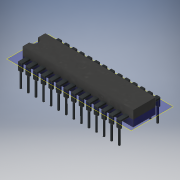
# Autodesk Inventor part: K572ПВ4
Saved by Autodesk Inventor 2019 (Build 230136000, 136)
## iProperties
Created: 2020-03-31
Part Number: K572ПВ4
Material: Generic
Document SubType Name: Modeling
Designer: user
Density: 1 g/cm^3
Appearance: Default
Author: user
Autodesk Inventor part; units mm, degrees
ref_plane "YZ Plane" through (0, 0, 0) normal (1, 0, 0) x (0, 1, 0)
ref_plane "XZ Plane" through (0, 0, 0) normal (0, 1, 0) x (-1, 0, 0)
ref_plane "XY Plane" through (0, 0, 0) normal (0, 0, 1) x (1, 0, 0)
sketch "Sketch1" plane through (0, 0, 0) normal (0, 1, 0) x (-1, 0, 0)
  line L0 (0, 0) -> (37, 0)
  line L1 (37, 0) -> (37, -7.5)
  line L2 (37, -7.5) -> (0, -7.5)
  line L3 (0, -7.5) -> (0, 0)
  dimension "d0" = 37
  dimension "d1" = 7.5
  constraints: 8 end point, 2 parallel, 1 horizontal, 1 perpendicular
  measures "d0" distance of L1.end L2.end
  measures "d1" distance between parallel lines of L0 L2
extrude "Extrusion1" add sketch "Sketch1" along normal blind 5
sketch "Sketch2" plane through (-37, 0, 0) normal (0, 0, 1) x (1, 0, 0)
  line L0 (37, 0) -> (37, 5) projected
  line L1 (2.6, 2.2) -> (1.4, 2.2)
  line L2 (1.4, 2.2) -> (1.4, 2.8)
  line L3 (1.4, 2.8) -> (2.6, 2.8)
  line L4 (2.6, 2.8) -> (2.6, 2.2)
  line L5 (2.6, 2.2) -> (1.4, 2.8) construction
  line L6 (1.4, 2.2) -> (2.6, 2.8) construction
  line L7 (5.14, 2.2) -> (3.94, 2.2)
  line L8 (3.94, 2.2) -> (3.94, 2.8)
  line L9 (3.94, 2.8) -> (5.14, 2.8)
  line L10 (5.14, 2.8) -> (5.14, 2.2)
  line L11 (7.68, 2.2) -> (6.48, 2.2)
  line L12 (6.48, 2.2) -> (6.48, 2.8)
  line L13 (6.48, 2.8) -> (7.68, 2.8)
  line L14 (7.68, 2.8) -> (7.68, 2.2)
  line L15 (10.22, 2.2) -> (9.02, 2.2)
  line L16 (9.02, 2.2) -> (9.02, 2.8)
  line L17 (9.02, 2.8) -> (10.22, 2.8)
  line L18 (10.22, 2.8) -> (10.22, 2.2)
  line L19 (12.76, 2.2) -> (11.56, 2.2)
  line L20 (11.56, 2.2) -> (11.56, 2.8)
  line L21 (11.56, 2.8) -> (12.76, 2.8)
  line L22 (12.76, 2.8) -> (12.76, 2.2)
  line L23 (15.3, 2.2) -> (14.1, 2.2)
  line L24 (14.1, 2.2) -> (14.1, 2.8)
  line L25 (14.1, 2.8) -> (15.3, 2.8)
  line L26 (15.3, 2.8) -> (15.3, 2.2)
  line L27 (17.84, 2.2) -> (16.64, 2.2)
  line L28 (16.64, 2.2) -> (16.64, 2.8)
  line L29 (16.64, 2.8) -> (17.84, 2.8)
  line L30 (17.84, 2.8) -> (17.84, 2.2)
  line L31 (20.38, 2.2) -> (19.18, 2.2)
  line L32 (19.18, 2.2) -> (19.18, 2.8)
  line L33 (19.18, 2.8) -> (20.38, 2.8)
  line L34 (20.38, 2.8) -> (20.38, 2.2)
  line L35 (22.92, 2.2) -> (21.72, 2.2)
  line L36 (21.72, 2.2) -> (21.72, 2.8)
  line L37 (21.72, 2.8) -> (22.92, 2.8)
  line L38 (22.92, 2.8) -> (22.92, 2.2)
  line L39 (25.46, 2.2) -> (24.26, 2.2)
  line L40 (24.26, 2.2) -> (24.26, 2.8)
  line L41 (24.26, 2.8) -> (25.46, 2.8)
  line L42 (25.46, 2.8) -> (25.46, 2.2)
  line L43 (28, 2.2) -> (26.8, 2.2)
  line L44 (26.8, 2.2) -> (26.8, 2.8)
  line L45 (26.8, 2.8) -> (28, 2.8)
  line L46 (28, 2.8) -> (28, 2.2)
  line L47 (30.54, 2.2) -> (29.34, 2.2)
  line L48 (29.34, 2.2) -> (29.34, 2.8)
  line L49 (29.34, 2.8) -> (30.54, 2.8)
  line L50 (30.54, 2.8) -> (30.54, 2.2)
  line L51 (33.08, 2.2) -> (31.88, 2.2)
  line L52 (31.88, 2.2) -> (31.88, 2.8)
  line L53 (31.88, 2.8) -> (33.08, 2.8)
  line L54 (33.08, 2.8) -> (33.08, 2.2)
  line L55 (35.62, 2.2) -> (34.42, 2.2)
  line L56 (34.42, 2.2) -> (34.42, 2.8)
  line L57 (34.42, 2.8) -> (35.62, 2.8)
  line L58 (35.62, 2.8) -> (35.62, 2.2)
  dimension "d19" = 1.2
  dimension "d20" = 0.6
  dimension "d21" = 1.2
  dimension "d22" = 0.6
  dimension "d23" = 1.2
  dimension "d25" = 1.2
  dimension "d27" = 1.2
  dimension "d28" = 0.6
  dimension "d29" = 1.2
  dimension "d31" = 1.2
  dimension "d32" = 0.6
  dimension "d33" = 1.2
  dimension "d34" = 0.6
  dimension "d35" = 1.2
  dimension "d36" = 0.6
  dimension "d37" = 1.2
  dimension "d38" = 0.6
  dimension "d39" = 1.2
  dimension "d40" = 0.6
  dimension "d41" = 1.2
  dimension "d42" = 0.6
  dimension "d43" = 1.2
  dimension "d44" = 0.6
  dimension "d45" = 1.2
  dimension "d46" = 0.6
  constraints: 116 end point, 28 parallel, 14 horizontal, 14 perpendicular
  measures "d19" distance of L2.end L3.end
  measures "d20" distance of L1.end L2.end
  measures "d21" distance of L9.start L9.end
  measures "d22" distance of L8.start L9.start
  measures "d23" distance of L13.start L13.end
  measures "d25" distance of L17.start L17.end
  measures "d27" distance of L21.start L21.end
  measures "d28" distance of L20.start L21.start
  measures "d29" distance of L25.start L25.end
  measures "d31" distance of L29.start L29.end
  measures "d32" distance of L28.start L29.start
  measures "d33" distance of L33.start L33.end
  measures "d34" distance of L32.start L33.start
  measures "d35" distance of L37.start L37.end
  measures "d36" distance of L36.start L37.start
  measures "d37" distance of L41.start L41.end
  measures "d38" distance of L40.start L41.start
  measures "d39" distance of L45.start L45.end
  measures "d40" distance of L44.start L45.start
  measures "d41" distance of L49.start L49.end
  measures "d42" distance of L48.start L49.start
  measures "d43" distance of L53.start L53.end
  measures "d44" distance of L52.start L53.start
  measures "d45" distance of L57.start L57.end
  measures "d46" distance of L56.start L57.start
extrude "Extrusion2" add sketch "Sketch2" along normal blind 3
sketch "Sketch3" plane through (0, 0, -7.5) normal (0, 0, -1) x (-1, 0, 0)
  line L0 (0, 0) -> (0, 5) projected
  line L1 (1.4, 2.2) -> (2.6, 2.2)
  line L2 (2.6, 2.2) -> (2.6, 2.8)
  line L3 (2.6, 2.8) -> (1.4, 2.8)
  line L4 (1.4, 2.8) -> (1.4, 2.2)
  line L5 (1.4, 2.2) -> (2.6, 2.8) construction
  line L6 (2.6, 2.2) -> (1.4, 2.8) construction
  line L7 (3.94, 2.2) -> (5.14, 2.2)
  line L8 (5.14, 2.2) -> (5.14, 2.8)
  line L9 (5.14, 2.8) -> (3.94, 2.8)
  line L10 (3.94, 2.8) -> (3.94, 2.2)
  line L11 (6.48, 2.2) -> (7.68, 2.2)
  line L12 (7.68, 2.2) -> (7.68, 2.8)
  line L13 (7.68, 2.8) -> (6.48, 2.8)
  line L14 (6.48, 2.8) -> (6.48, 2.2)
  line L15 (9.02, 2.2) -> (10.22, 2.2)
  line L16 (10.22, 2.2) -> (10.22, 2.8)
  line L17 (10.22, 2.8) -> (9.02, 2.8)
  line L18 (9.02, 2.8) -> (9.02, 2.2)
  line L19 (11.56, 2.2) -> (12.76, 2.2)
  line L20 (12.76, 2.2) -> (12.76, 2.8)
  line L21 (12.76, 2.8) -> (11.56, 2.8)
  line L22 (11.56, 2.8) -> (11.56, 2.2)
  line L23 (14.1, 2.2) -> (15.3, 2.2)
  line L24 (15.3, 2.2) -> (15.3, 2.8)
  line L25 (15.3, 2.8) -> (14.1, 2.8)
  line L26 (14.1, 2.8) -> (14.1, 2.2)
  line L27 (16.64, 2.2) -> (17.84, 2.2)
  line L28 (17.84, 2.2) -> (17.84, 2.8)
  line L29 (17.84, 2.8) -> (16.64, 2.8)
  line L30 (16.64, 2.8) -> (16.64, 2.2)
  line L31 (16.64, 2.8) -> (16.64, 2.2)
  line L32 (17.84, 2.8) -> (16.64, 2.8)
  line L33 (17.84, 2.2) -> (17.84, 2.8)
  line L34 (16.64, 2.2) -> (17.84, 2.2)
  line L35 (19.18, 2.8) -> (19.18, 2.2)
  line L36 (20.38, 2.8) -> (19.18, 2.8)
  line L37 (20.38, 2.2) -> (20.38, 2.8)
  line L38 (19.18, 2.2) -> (20.38, 2.2)
  line L39 (21.72, 2.8) -> (21.72, 2.2)
  line L40 (22.92, 2.8) -> (21.72, 2.8)
  line L41 (22.92, 2.2) -> (22.92, 2.8)
  line L42 (21.72, 2.2) -> (22.92, 2.2)
  line L43 (24.26, 2.8) -> (24.26, 2.2)
  line L44 (25.46, 2.8) -> (24.26, 2.8)
  line L45 (25.46, 2.2) -> (25.46, 2.8)
  line L46 (24.26, 2.2) -> (25.46, 2.2)
  line L47 (26.8, 2.8) -> (26.8, 2.2)
  line L48 (28, 2.8) -> (26.8, 2.8)
  line L49 (28, 2.2) -> (28, 2.8)
  line L50 (26.8, 2.2) -> (28, 2.2)
  line L51 (29.34, 2.8) -> (29.34, 2.2)
  line L52 (30.54, 2.8) -> (29.34, 2.8)
  line L53 (30.54, 2.2) -> (30.54, 2.8)
  line L54 (29.34, 2.2) -> (30.54, 2.2)
  line L55 (31.88, 2.8) -> (31.88, 2.2)
  line L56 (33.08, 2.8) -> (31.88, 2.8)
  line L57 (33.08, 2.2) -> (33.08, 2.8)
  line L58 (31.88, 2.2) -> (33.08, 2.2)
  line L59 (34.42, 2.8) -> (34.42, 2.2)
  line L60 (35.62, 2.8) -> (34.42, 2.8)
  line L61 (35.62, 2.2) -> (35.62, 2.8)
  line L62 (34.42, 2.2) -> (35.62, 2.2)
  dimension "d63" = 1.2
  dimension "d64" = 0.6
  dimension "d65" = 1.2
  dimension "d66" = 0.6
  dimension "d67" = 1.2
  dimension "d68" = 0.6
  dimension "d69" = 1.2
  dimension "d70" = 0.6
  dimension "d71" = 1.2
  dimension "d72" = 0.6
  dimension "d73" = 1.2
  dimension "d74" = 0.6
  dimension "d75" = 1.2
  dimension "d76" = 0.6
  dimension "d77" = 1.2
  dimension "d78" = 0.6
  dimension "d79" = 1.2
  dimension "d80" = 0.6
  dimension "d81" = 1.2
  dimension "d82" = 0.6
  dimension "d83" = 1.2
  dimension "d84" = 0.6
  dimension "d85" = 1.2
  dimension "d86" = 0.6
  dimension "d87" = 1.2
  dimension "d88" = 0.6
  dimension "d89" = 1.2
  dimension "d90" = 0.6
  dimension "d91" = 1.2
  dimension "d92" = 0.6
  constraints: 124 end point, 30 parallel, 15 horizontal, 15 perpendicular
  measures "d63" distance of L3.end L2.end
  measures "d64" distance between parallel lines of L1 L3
  measures "d65" distance of L10.start L9.start
  measures "d66" distance between parallel lines of L7 L9
  measures "d67" distance of L14.start L13.start
  measures "d68" distance between parallel lines of L11 L13
  measures "d69" distance of L18.start L17.start
  measures "d70" distance between parallel lines of L15 L17
  measures "d71" distance of L22.start L21.start
  measures "d72" distance between parallel lines of L19 L21
  measures "d73" distance of L26.start L25.start
  measures "d74" distance between parallel lines of L23 L25
  measures "d75" distance of L30.start L29.start
  measures "d76" distance between parallel lines of L27 L29
  measures "d77" distance of L32.end L32.start
  measures "d78" distance between parallel lines of L34 L32
  measures "d79" distance of L36.end L36.start
  measures "d80" distance between parallel lines of L38 L36
  measures "d81" distance of L40.end L40.start
  measures "d82" distance between parallel lines of L42 L40
  measures "d83" distance of L44.end L44.start
  measures "d84" distance between parallel lines of L46 L44
  measures "d85" distance of L48.end L48.start
  measures "d86" distance between parallel lines of L50 L48
  measures "d87" distance of L52.end L52.start
  measures "d88" distance between parallel lines of L54 L52
  measures "d89" distance of L56.end L56.start
  measures "d90" distance between parallel lines of L58 L56
  measures "d91" distance of L60.end L60.start
  measures "d92" distance between parallel lines of L62 L60
extrude "Extrusion3" add sketch "Sketch3" along normal blind 3
ref_plane "Work Plane2" through (-35.6, 2.2, 3) normal (0, -1, 0) x (1, 0, 0)
sketch "Sketch6" plane through (-35.6, 2.2, 3) normal (0, -1, 0) x (1, 0, 0)
  line L0 (0, 0) -> (1.2, 0)
  line L1 (1.2, 0) -> (1.2, -0.6)
  line L2 (1.2, -0.6) -> (0, -0.6)
  line L3 (0, -0.6) -> (0, 0)
  line L4 (2.5041, 0) -> (3.7041, 0)
  line L5 (3.7041, 0) -> (3.7041, -0.6)
  line L6 (3.7041, -0.6) -> (2.5041, -0.6)
  line L7 (2.5041, -0.6) -> (2.5041, 0)
  line L8 (5.0877, 0) -> (6.2877, 0)
  line L9 (6.2877, 0) -> (6.2877, -0.6)
  line L10 (6.2877, -0.6) -> (5.0877, -0.6)
  line L11 (5.0877, -0.6) -> (5.0877, 0)
  line L12 (7.6344, 0) -> (8.8344, 0)
  line L13 (8.8344, 0) -> (8.8344, -0.6)
  line L14 (8.8344, -0.6) -> (7.6344, -0.6)
  line L15 (7.6344, -0.6) -> (7.6344, 0)
  line L16 (10.1527, 0) -> (11.3527, 0)
  line L17 (11.3527, 0) -> (11.3527, -0.6)
  line L18 (11.3527, -0.6) -> (10.1527, -0.6)
  line L19 (10.1527, -0.6) -> (10.1527, 0)
  line L20 (12.7058, 0) -> (13.9058, 0)
  line L21 (13.9058, 0) -> (13.9058, -0.6)
  line L22 (13.9058, -0.6) -> (12.7058, -0.6)
  line L23 (12.7058, -0.6) -> (12.7058, 0)
  line L24 (15.2415, 0) -> (16.4415, 0)
  line L25 (16.4415, 0) -> (16.4415, -0.6)
  line L26 (16.4415, -0.6) -> (15.2415, -0.6)
  line L27 (15.2415, -0.6) -> (15.2415, 0)
  line L28 (17.7945, 0) -> (18.9945, 0)
  line L29 (18.9945, 0) -> (18.9945, -0.6)
  line L30 (18.9945, -0.6) -> (17.7945, -0.6)
  line L31 (17.7945, -0.6) -> (17.7945, 0)
  line L32 (20.3302, 0) -> (21.5302, 0)
  line L33 (21.5302, 0) -> (21.5302, -0.6)
  line L34 (21.5302, -0.6) -> (20.3302, -0.6)
  line L35 (20.3302, -0.6) -> (20.3302, 0)
  line L36 (22.8658, 0) -> (24.0658, 0)
  line L37 (24.0658, 0) -> (24.0658, -0.6)
  line L38 (24.0658, -0.6) -> (22.8658, -0.6)
  line L39 (22.8658, -0.6) -> (22.8658, 0)
  line L40 (-0.0033, -12.9) -> (1.1967, -12.9)
  line L41 (1.1967, -12.9) -> (1.1967, -13.5)
  line L42 (1.1967, -13.5) -> (-0.0033, -13.5)
  line L43 (-0.0033, -13.5) -> (-0.0033, -12.9)
  line L44 (25.3789, 0) -> (26.5789, 0)
  line L45 (26.5789, 0) -> (26.5789, -0.6)
  line L46 (26.5789, -0.6) -> (25.3789, -0.6)
  line L47 (25.3789, -0.6) -> (25.3789, 0)
  line L48 (27.932, 0) -> (29.132, 0)
  line L49 (29.132, 0) -> (29.132, -0.6)
  line L50 (29.132, -0.6) -> (27.932, -0.6)
  line L51 (27.932, -0.6) -> (27.932, 0)
  line L52 (30.4676, 0) -> (31.6676, 0)
  line L53 (31.6676, 0) -> (31.6676, -0.6)
  line L54 (31.6676, -0.6) -> (30.4676, -0.6)
  line L55 (30.4676, -0.6) -> (30.4676, 0)
  line L56 (33.0033, 0) -> (34.2033, 0)
  line L57 (34.2033, 0) -> (34.2033, -0.6)
  line L58 (34.2033, -0.6) -> (33.0033, -0.6)
  line L59 (33.0033, -0.6) -> (33.0033, 0)
  line L60 (2.5008, -12.9) -> (3.7008, -12.9)
  line L61 (3.7008, -12.9) -> (3.7008, -13.5)
  line L62 (3.7008, -13.5) -> (2.5008, -13.5)
  line L63 (2.5008, -13.5) -> (2.5008, -12.9)
  line L64 (5.0844, -12.9) -> (6.2844, -12.9)
  line L65 (6.2844, -12.9) -> (6.2844, -13.5)
  line L66 (6.2844, -13.5) -> (5.0844, -13.5)
  line L67 (5.0844, -13.5) -> (5.0844, -12.9)
  line L68 (7.6311, -12.9) -> (8.8311, -12.9)
  line L69 (8.8311, -12.9) -> (8.8311, -13.5)
  line L70 (8.8311, -13.5) -> (7.6311, -13.5)
  line L71 (7.6311, -13.5) -> (7.6311, -12.9)
  line L72 (10.1494, -12.9) -> (11.3494, -12.9)
  line L73 (11.3494, -12.9) -> (11.3494, -13.5)
  line L74 (11.3494, -13.5) -> (10.1494, -13.5)
  line L75 (10.1494, -13.5) -> (10.1494, -12.9)
  line L76 (12.7025, -12.9) -> (13.9025, -12.9)
  line L77 (13.9025, -12.9) -> (13.9025, -13.5)
  line L78 (13.9025, -13.5) -> (12.7025, -13.5)
  line L79 (12.7025, -13.5) -> (12.7025, -12.9)
  line L80 (15.2382, -12.9) -> (16.4382, -12.9)
  line L81 (16.4382, -12.9) -> (16.4382, -13.5)
  line L82 (16.4382, -13.5) -> (15.2382, -13.5)
  line L83 (15.2382, -13.5) -> (15.2382, -12.9)
  line L84 (17.7912, -12.9) -> (18.9912, -12.9)
  line L85 (18.9912, -12.9) -> (18.9912, -13.5)
  line L86 (18.9912, -13.5) -> (17.7912, -13.5)
  line L87 (17.7912, -13.5) -> (17.7912, -12.9)
  line L88 (20.3269, -12.9) -> (21.5269, -12.9)
  line L89 (21.5269, -12.9) -> (21.5269, -13.5)
  line L90 (21.5269, -13.5) -> (20.3269, -13.5)
  line L91 (20.3269, -13.5) -> (20.3269, -12.9)
  line L92 (22.8625, -12.9) -> (24.0625, -12.9)
  line L93 (24.0625, -12.9) -> (24.0625, -13.5)
  line L94 (24.0625, -13.5) -> (22.8625, -13.5)
  line L95 (22.8625, -13.5) -> (22.8625, -12.9)
  line L96 (25.3756, -13.5) -> (25.3756, -12.9)
  line L97 (25.3756, -12.9) -> (26.5756, -12.9)
  line L98 (26.5756, -13.5) -> (25.3756, -13.5)
  line L99 (26.5756, -12.9) -> (26.5756, -13.5)
  line L100 (27.9287, -13.5) -> (27.9287, -12.9)
  line L101 (27.9287, -12.9) -> (29.1287, -12.9)
  line L102 (29.1287, -13.5) -> (27.9287, -13.5)
  line L103 (29.1287, -12.9) -> (29.1287, -13.5)
  line L104 (30.4643, -13.5) -> (30.4643, -12.9)
  line L105 (30.4643, -12.9) -> (31.6643, -12.9)
  line L106 (31.6643, -13.5) -> (30.4643, -13.5)
  line L107 (31.6643, -12.9) -> (31.6643, -13.5)
  line L108 (33, -13.5) -> (33, -12.9)
  line L109 (34.2, -12.9) -> (34.2, -13.5)
  line L110 (34.2, -13.5) -> (33, -13.5)
  line L111 (33, -12.9) -> (34.2, -12.9)
  point P0 (35.6, -3)
  dimension "d127" = 1.2
  dimension "d128" = 0.6
  dimension "d129" = 1.2
  dimension "d130" = 0.6
  dimension "d131" = 1.2
  dimension "d132" = 0.6
  dimension "d133" = 1.2
  dimension "d134" = 0.6
  dimension "d135" = 1.2
  dimension "d136" = 0.6
  dimension "d137" = 1.2
  dimension "d138" = 0.6
  dimension "d139" = 1.2
  dimension "d140" = 0.6
  dimension "d141" = 1.2
  dimension "d142" = 0.6
  dimension "d143" = 1.2
  dimension "d144" = 0.6
  dimension "d145" = 1.2
  dimension "d146" = 0.6
  dimension "d152" = 1.2
  dimension "d153" = 0.6
  dimension "d154" = 1.2
  dimension "d155" = 0.6
  dimension "d156" = 1.2
  dimension "d157" = 0.6
  dimension "d158" = 1.2
  dimension "d159" = 0.6
  dimension "d160" = 1.2
  dimension "d161" = 0.6
  dimension "d162" = 1.2
  dimension "d163" = 0.6
  dimension "d164" = 1.2
  dimension "d165" = 0.6
  dimension "d166" = 1.2
  dimension "d167" = 0.6
  dimension "d168" = 1.2
  dimension "d169" = 0.6
  dimension "d170" = 1.2
  dimension "d171" = 0.6
  dimension "d172" = 1.2
  dimension "d173" = 0.6
  dimension "d174" = 1.2
  dimension "d175" = 0.6
  dimension "d176" = 1.2
  dimension "d177" = 0.6
  dimension "d178" = 1.2
  dimension "d179" = 0.6
  dimension "d180" = 1.2
  dimension "d181" = 0.6
  dimension "d182" = 1.2
  dimension "d183" = 0.6
  dimension "d184" = 1.2
  dimension "d185" = 0.6
  dimension "d186" = 1.2
  dimension "d187" = 0.6
  constraints: 224 end point, 56 parallel, 28 horizontal, 28 perpendicular
  measures "d127" distance of L1.end L2.end
  measures "d128" distance of L0.end L1.end
  measures "d129" distance of L5.end L6.end
  measures "d130" distance of L4.end L5.end
  measures "d131" distance of L9.end L10.end
  measures "d132" distance of L8.end L9.end
  measures "d133" distance of L13.end L14.end
  measures "d134" distance of L12.end L13.end
  measures "d135" distance of L17.end L18.end
  measures "d136" distance of L16.end L17.end
  measures "d137" distance of L21.end L22.end
  measures "d138" distance of L20.end L21.end
  measures "d139" distance of L25.end L26.end
  measures "d140" distance of L24.end L25.end
  measures "d141" distance of L29.end L30.end
  measures "d142" distance of L28.end L29.end
  measures "d143" distance of L33.end L34.end
  measures "d144" distance of L32.end L33.end
  measures "d145" distance of L37.end L38.end
  measures "d146" distance of L36.end L37.end
  measures "d152" distance of L41.end L42.end
  measures "d153" distance of L40.end L41.end
  measures "d154" distance of L46.start L47.start
  measures "d155" distance of L44.end L46.start
  measures "d156" distance of L50.start L51.start
  measures "d157" distance of L48.end L50.start
  measures "d158" distance of L54.start L55.start
  measures "d159" distance of L52.end L54.start
  measures "d160" distance of L57.end L59.start
  measures "d161" distance of L57.start L57.end
  measures "d162" distance of L61.end L62.end
  measures "d163" distance of L61.start L61.end
  measures "d164" distance of L65.end L67.start
  measures "d165" distance of L64.end L65.end
  measures "d166" distance of L69.end L71.start
  measures "d167" distance of L69.start L69.end
  measures "d168" distance of L73.end L75.start
  measures "d169" distance of L72.end L73.end
  measures "d170" distance of L77.end L79.start
  measures "d171" distance of L77.start L77.end
  measures "d172" distance of L81.end L83.start
  measures "d173" distance of L81.start L81.end
  measures "d174" distance of L86.start L87.start
  measures "d175" distance of L84.end L86.start
  measures "d176" distance of L90.start L91.start
  measures "d177" distance of L89.start L90.start
  measures "d178" distance of L94.start L95.start
  measures "d179" distance of L92.end L94.start
  measures "d180" distance of L98.start L96.start
  measures "d181" distance of L99.start L98.start
  measures "d182" distance of L102.start L100.start
  measures "d183" distance of L101.end L102.start
  measures "d184" distance of L106.start L104.start
  measures "d185" distance of L105.end L106.start
  measures "d186" distance of L110.start L110.end
  measures "d187" distance of L109.start L110.start
extrude "Extrusion6" add sketch "Sketch6" along normal blind 2
sketch "Sketch7" plane through (-35.6, 0.2, 3) normal (0, -1, 0) x (1, 0, 0)
  line L0 (1.2, 0) -> (0, 0) projected
  line L1 (0.6, 0) -> (0.6, -0.6)
  line L2 (1.2, -0.6) -> (0, -0.6) projected
  circle A0 centre (0.6, -0.3) radius 0.3
  circle A1 centre (3.1041, -0.3) radius 0.3
  circle A2 centre (5.6839, -0.3) radius 0.3
  circle A3 centre (8.2344, -0.3) radius 0.3
  line L3 (7.6344, -0.6) -> (8.8344, -0.6) projected
  circle A4 centre (10.7564, -0.3) radius 0.3
  line L4 (11.3564, -0.6) -> (10.1564, -0.6) projected
  circle A5 centre (13.3029, -0.3) radius 0.3
  circle A6 centre (15.8415, -0.3) radius 0.3
  circle A7 centre (18.3872, -0.3) radius 0.3
  circle A8 centre (20.9251, -0.3) radius 0.3
  circle A9 centre (23.4572, -0.3) radius 0.3
  circle A10 centre (26.0037, -0.3) radius 0.3
  circle A11 centre (28.5423, -0.3) radius 0.3
  circle A12 centre (31.0881, -0.3) radius 0.3
  circle A13 centre (33.6259, -0.3) radius 0.3
  line L5 (0.5887, -12.8982) -> (0.5887, -13.4982)
  circle A14 centre (0.5887, -13.1982) radius 0.3
  circle A15 centre (3.0928, -13.1982) radius 0.3
  circle A16 centre (5.6726, -13.1982) radius 0.3
  circle A17 centre (8.2231, -13.1982) radius 0.3
  circle A18 centre (10.7451, -13.1982) radius 0.3
  circle A19 centre (13.2916, -13.1982) radius 0.3
  circle A20 centre (15.8301, -13.1982) radius 0.3
  circle A21 centre (18.3759, -13.1982) radius 0.3
  circle A22 centre (20.9138, -13.1982) radius 0.3
  circle A23 centre (25.9924, -13.1982) radius 0.3
  circle A24 centre (28.531, -13.1982) radius 0.3
  circle A25 centre (31.0768, -13.1982) radius 0.3
  circle A26 centre (33.6146, -13.1982) radius 0.3
  circle A27 centre (23.4459, -13.1982) radius 0.3
  point P0 (35.6, -3)
  point P1 (11.3527, -0.6)
  point P2 (10.16, -0.6)
  dimension "d149" = 0.6
  dimension "d188" = 0.6
  dimension "d189" = 0.6
  dimension "d190" = 0.6
  dimension "d191" = 0.6
  dimension "d192" = 0.6
  constraints: 28 centre point, 4 end point, 4 midpoint, 2 tangent
  measures "d149" diameter of A0
  measures "d188" diameter of A1
  measures "d189" diameter of A2
  measures "d190" diameter of A14
  measures "d191" diameter of A15
  measures "d192" diameter of A16
extrude "Extrusion7" add sketch "Sketch7" along normal blind 5
sketch "Sketch8" plane through (0, 5, 0) normal (0, 1, 0) x (1, 0, 0)
  point P0 (0, 0)
  point P1 (-37, 3.6184)
hole "Hole1" at (-37, 5, -3.6184) direction (0, -1, 0) diameter 3 depth 2.2875
body "Solid1"
